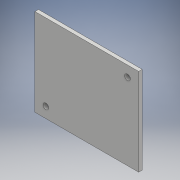
# Autodesk Inventor part: Lid
Saved by Autodesk Inventor 2017 (Build 210142000, 142)
## iProperties
Created: 2017-03-21
Part Number: Lid
Material: Generic
Document SubType Name: Modeling
Designer: Liam
Density: 1 g/cm^3
Appearance: Default
Author: Liam
Autodesk Inventor part; units mm, degrees
ref_plane "YZ Plane" through (0, 0, 0) normal (1, 0, 0) x (0, 1, 0)
ref_plane "XZ Plane" through (0, 0, 0) normal (0, 1, 0) x (-1, 0, 0)
ref_plane "XY Plane" through (0, 0, 0) normal (0, 0, 1) x (1, 0, 0)
sketch "Sketch1" plane through (0, 0, 0) normal (0, 1, 0) x (-1, 0, 0)
  line L0 (0, 0) -> (72.9, 0)
  line L1 (72.9, 0) -> (72.9, -61.3)
  line L2 (72.9, -61.3) -> (0, -61.3)
  line L3 (0, -61.3) -> (0, 0)
  dimension "d0" = 72.9
  dimension "d1" = 61.3
  constraints: 8 end point, 2 parallel, 1 horizontal, 1 perpendicular
  measures "d0" distance of L1.end L2.end
  measures "d1" distance of L0.end L1.end
extrude "Extrusion1" add sketch "Sketch1" along normal blind 2.5
sketch "Sketch2" plane through (0, 2.5, 0) normal (0, 1, 0) x (1, 0, 0)
  line L0 (-72.9, 0) -> (0, 0) projected
  line L1 (-72.9, 61.3) -> (-72.9, 0) projected
  line L2 (0, 61.3) -> (-72.9, 61.3) projected
  line L3 (0, 0) -> (0, 61.3) projected
  point P0 (-65.2, 53.8)
  point P1 (-7.8, 7.5)
  dimension "d6" = 7.7
  dimension "d7" = 7.5
  dimension "d8" = 7.5
  dimension "d9" = 7.8
  measures "d6" distance from line of point (-65.2, 53.8) L1
  measures "d7" distance from line of L2 point (-65.2, 53.8)
  measures "d8" distance from line of L0 point (-7.8, 7.5)
  measures "d9" distance from line of point (-7.8, 7.5) L3
hole "Hole1" at (-65.2, 2.5, -53.8) at (-7.8, 2.5, -7.5) direction (0, -1, 0) diameter 4 end through all
sketch "Sketch3" plane through (0, 2.5, 0) normal (0, 1, 0) x (1, 0, 0)
  line L0 (-57.9, 38.9915) -> (-15.0143, 38.9915) construction
  line L1 (-15.0143, 38.9915) -> (-15.0143, 22.3) construction
  line L2 (-15.0143, 22.3) -> (-57.9, 22.3) construction
  line L3 (-57.9, 22.3) -> (-57.9, 38.9915) construction
  line L4 (-72.9, 61.3) -> (-72.9, 0) projected
  line L5 (-72.9, 0) -> (0, 0) projected
  spline S0 degree 2 poles (-52.0066, 22.2116) (-54.2985, 22.2116) (-56.7541, 24.9537) (-56.7677, 27.6003) knots 0 0 0 1 2 2 2
  line L6 (-56.7677, 27.6003) -> (-56.7677, 29.0873)
  spline S1 degree 2 poles (-56.7677, 29.0873) (-56.7677, 31.843) (-54.3803, 34.9671) (-52.2248, 34.9671) knots 0 0 0 1 2 2 2
  spline S2 degree 2 poles (-52.2248, 34.9671) (-50.0694, 34.9671) (-47.9275, 32.2114) (-47.9139, 29.3056) knots 0 0 0 1 2 2 2
  line L7 (-47.9139, 29.3056) -> (-47.9139, 27.9823)
  line L8 (-47.9139, 27.9823) -> (-54.7759, 27.9823)
  line L9 (-54.7759, 27.9823) -> (-54.7759, 27.6958)
  spline S3 degree 2 poles (-54.7759, 27.6958) (-54.7759, 25.7177) (-53.2889, 23.9305) (-51.8838, 23.9305) knots 0 0 0 1 2 2 2
  spline S4 degree 2 poles (-51.8838, 23.9305) (-50.997, 23.9305) (-49.6465, 24.599) (-49.0598, 25.3221) knots 0 0 0 1 2 2 2
  line L10 (-49.0598, 25.3221) -> (-48.0094, 24.0533)
  spline S5 degree 2 poles (-48.0094, 24.0533) (-49.319, 22.2116) (-52.0066, 22.2116) knots 0 0 0 1 1 1
  spline S6 degree 2 poles (-52.2248, 33.2345) (-53.4799, 33.2345) (-54.6804, 31.5156) (-54.7623, 29.7148) knots 0 0 0 1 2 2 2
  line L11 (-54.7623, 29.7148) -> (-49.9193, 29.7148)
  line L12 (-49.9193, 29.7148) -> (-49.9193, 29.9877)
  spline S7 degree 2 poles (-49.9193, 29.9877) (-50.0012, 31.7339) (-51.1062, 33.2345) (-52.2248, 33.2345) knots 0 0 0 1 2 2 2
  line L13 (-34.3808, 22.4435) -> (-36.4817, 22.4435)
  line L14 (-36.4817, 22.4435) -> (-36.4817, 30.0832)
  line L15 (-36.4817, 30.0832) -> (-43.1391, 30.0832)
  line L16 (-43.1391, 30.0832) -> (-43.1391, 22.4435)
  line L17 (-43.1391, 22.4435) -> (-45.2127, 22.4435)
  line L18 (-45.2127, 22.4435) -> (-45.2127, 38.9915)
  line L19 (-45.2127, 38.9915) -> (-43.1391, 38.9915)
  line L20 (-43.1391, 38.9915) -> (-43.1391, 31.8703)
  line L21 (-43.1391, 31.8703) -> (-36.4817, 31.8703)
  line L22 (-36.4817, 31.8703) -> (-36.4817, 38.9915)
  line L23 (-36.4817, 38.9915) -> (-34.3808, 38.9915)
  line L24 (-34.3808, 38.9915) -> (-34.3808, 22.4435)
  line L25 (-28.6102, 22.4435) -> (-30.6974, 22.4435)
  line L26 (-30.6974, 22.4435) -> (-30.6974, 38.9915)
  line L27 (-30.6974, 38.9915) -> (-28.6102, 38.9915)
  line L28 (-28.6102, 38.9915) -> (-28.6102, 22.4435)
  line L29 (-15.2817, 37.2044) -> (-19.6336, 37.2044)
  line L30 (-19.6336, 37.2044) -> (-19.6336, 22.4435)
  line L31 (-19.6336, 22.4435) -> (-21.7209, 22.4435)
  line L32 (-21.7209, 22.4435) -> (-21.7209, 37.2044)
  line L33 (-21.7209, 37.2044) -> (-26.0591, 37.2044)
  line L34 (-26.0591, 37.2044) -> (-26.0591, 38.9915)
  line L35 (-26.0591, 38.9915) -> (-15.2817, 38.9915)
  line L36 (-15.2817, 38.9915) -> (-15.2817, 37.2044)
  dimension "d17" = 42.8857
  dimension "d18" = 15
  dimension "d19" = 16.6915
  dimension "d20" = 22.3
  constraints: 2 other
  measures "d17" distance between parallel lines of L1 L3
  measures "d18" distance between parallel lines of L3 L4
  measures "d19" distance between parallel lines of L0 L2
  measures "d20" distance between parallel lines of L5 L2
extrude "Extrusion2" add sketch "Sketch3" along normal blind 2
body "Solid1"
